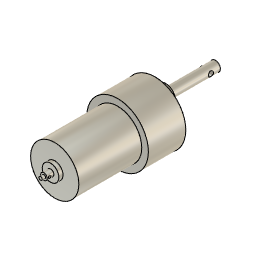
Motor v3 (Autodesk Fusion 360 design; units mm, degrees)
Autodesk Fusion 360 part; units mm, degrees
sketch "Sketch1" plane through (0, 0, 0) normal (0, 1, 0) x (1, 0, 0)
  circle A0 centre (0, 0) radius 14.5
  dimension "d1" = 29
  constraint coincident A0.centre origin
  measures "d1" diameter of A0
extrude "Extrude1" add sketch "Sketch1" along normal blind 37.8
sketch "Sketch2" plane through (0, 37.8, 0) normal (0, 1, 0) x (-1, 0, 0)
  circle A0 centre (0, 0) radius 14.5
  circle A1 centre (0, 0) radius 18.5
  dimension "d4" = 37
  constraint coincident A0.centre A1.centre
  measures "d4" diameter of A1
extrude "Extrude2" add sketch "Sketch2" along normal blind 22.5 contours A0 | A1
sketch "Sketch3" plane through (0, 60.3, 0) normal (0, 1, 0) x (-1, 0, 0)
  circle A0 centre (0, 0) radius 18.5
  circle A1 centre (0, 6) radius 6
  dimension "d7" = 12
  measures "d7" diameter of A1
extrude "Extrude3" add sketch "Sketch3" along normal blind 6.3 contours A1
sketch "Sketch4" plane through (0, 66.6, 0) normal (0, 1, 0) x (-1, 0, 0)
  circle A0 centre (0, 6) radius 6
  circle A1 centre (0, 6) radius 3
  dimension "d10" = 6
  constraint concentric A0 A1
  measures "d10" diameter of A1
extrude "Extrude4" add sketch "Sketch4" along normal blind 30 contours A1
sketch "Sketch5" plane through (0, 0, 0) normal (1, 0, 0) x (0, 1, 0)
sketch "Sketch6" plane through (0, 0, 0) normal (1, 0, 0) x (0, 1, 0)
  circle A0 centre (91, 6) radius 1.5
  dimension "d13" = 3
  measures "d13" diameter of A0
extrude "Extrude5" cut sketch "Sketch6" along normal mid plane 6
sketch "Sketch7" plane through (0, 0, 0) normal (0, -1, 0) x (1, 0, 0)
  circle A0 centre (0, 0) radius 14.5
  circle A1 centre (0, 0) radius 5
  dimension "d16" = 10
  constraint concentric A0 A1
  measures "d16" diameter of A1
extrude "Extrude6" add sketch "Sketch7" along normal blind 2.5 contours A1
sketch "Sketch8" plane through (0, -2.5, 0) normal (0, -1, 0) x (1, 0, 0)
  circle A0 centre (0, 0) radius 5
  circle A1 centre (0, 0) radius 2
  dimension "d19" = 4
  constraint coincident A0.centre A1.centre
  measures "d19" diameter of A1
extrude "Extrude7" add sketch "Sketch8" along normal blind 4 contours A1
sketch "Sketch9" plane through (0, -6.5, 0) normal (0, -1, 0) x (1, 0, 0)
  circle A0 centre (0, 0) radius 2
  circle A1 centre (0, 0) radius 1
  dimension "d22" = 2
  constraint coincident A0.centre A1.centre
  measures "d22" diameter of A1
extrude "Extrude8" add sketch "Sketch9" along normal blind 2 contours A1
sketch "Sketch10" plane through (0, 0, 0) normal (1, 0, 0) x (0, 1, 0)
  circle A0 centre (-5, 0) radius 0.75
  dimension "d25" = 1.5
  measures "d25" diameter of A0
extrude "Extrude9" cut sketch "Sketch10" along normal mid plane 5
